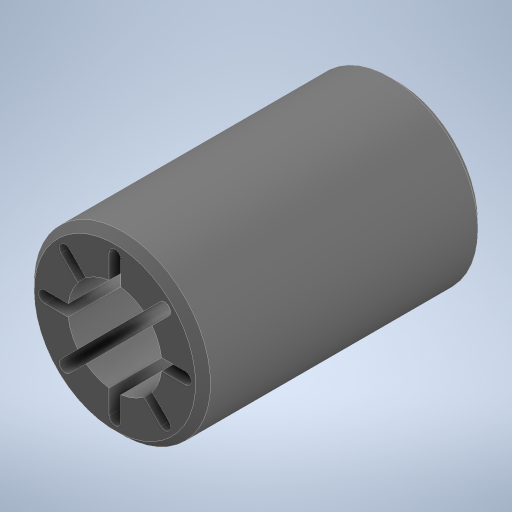
# Autodesk Inventor part: Dry Bearing
Saved by Autodesk Inventor 2023 (Build 270158000, 158)
## iProperties
Created: 2023-02-06
Part Number: Dry Bearing
Material: Generic
Document SubType Name: Modeling
Designer: mbear
Density: 1 g/cm^3
Appearance: Gray
Author: mbear
Autodesk Inventor part; units mm, degrees
ref_plane "YZ Plane" through (0, 0, 0) normal (1, 0, 0) x (0, 1, 0)
ref_plane "XZ Plane" through (0, 0, 0) normal (0, 1, 0) x (-1, 0, 0)
ref_plane "XY Plane" through (0, 0, 0) normal (0, 0, 1) x (1, 0, 0)
sketch "Sketch1" plane through (0, 0, 0) normal (0, 0, 1) x (1, 0, 0)
  circle A0 centre (0, 0) radius 7.5
  circle A1 centre (0, 0) radius 4
  dimension "d0" = 15
  dimension "d1" = 8
  constraints: 2 centre point, 2 coincident
  measures "d0" diameter of A0
  measures "d1" diameter of A1
extrude "Extrusion1" add sketch "Sketch1" along normal blind 24
sketch "Sketch2" plane through (0, 0, 24) normal (0, 0, 1) x (1, 0, 0)
  arc A0 (0.5, 6) -> (-0.5, 6) centre (0, 6) ccw
  line L0 (-0.5, 6) -> (-0.5, 2.6094)
  line L1 (-0.5, 2.6094) -> (0.5, 2.6094)
  line L2 (0.5, 2.6094) -> (0.5, 6)
  line L3 (-4.5962, 3.8891) -> (-2.1987, 1.4916)
  arc A1 (-3.8891, 4.5962) -> (-4.5962, 3.8891) centre (-4.2426, 4.2426) ccw
  line L4 (-1.4916, 2.1987) -> (-3.8891, 4.5962)
  line L5 (-2.1987, 1.4916) -> (-1.4916, 2.1987)
  line L6 (-6, -0.5) -> (-2.6094, -0.5)
  arc A2 (-6, 0.5) -> (-6, -0.5) centre (-6, 0) ccw
  line L7 (-2.6094, 0.5) -> (-6, 0.5)
  line L8 (-2.6094, -0.5) -> (-2.6094, 0.5)
  line L9 (-3.8891, -4.5962) -> (-1.4916, -2.1987)
  arc A3 (-4.5962, -3.8891) -> (-3.8891, -4.5962) centre (-4.2426, -4.2426) ccw
  line L10 (-2.1987, -1.4916) -> (-4.5962, -3.8891)
  line L11 (-1.4916, -2.1987) -> (-2.1987, -1.4916)
  line L12 (0.5, -6) -> (0.5, -2.6094)
  arc A4 (-0.5, -6) -> (0.5, -6) centre (0, -6) ccw
  line L13 (-0.5, -2.6094) -> (-0.5, -6)
  line L14 (0.5, -2.6094) -> (-0.5, -2.6094)
  line L15 (4.5962, -3.8891) -> (2.1987, -1.4916)
  arc A5 (3.8891, -4.5962) -> (4.5962, -3.8891) centre (4.2426, -4.2426) ccw
  line L16 (1.4916, -2.1987) -> (3.8891, -4.5962)
  line L17 (2.1987, -1.4916) -> (1.4916, -2.1987)
  line L18 (6, 0.5) -> (2.6094, 0.5)
  arc A6 (6, -0.5) -> (6, 0.5) centre (6, 0) ccw
  line L19 (2.6094, -0.5) -> (6, -0.5)
  line L20 (2.6094, 0.5) -> (2.6094, -0.5)
  line L21 (3.8891, 4.5962) -> (1.4916, 2.1987)
  arc A7 (4.5962, 3.8891) -> (3.8891, 4.5962) centre (4.2426, 4.2426) ccw
  line L22 (2.1987, 1.4916) -> (4.5962, 3.8891)
  line L23 (1.4916, 2.1987) -> (2.1987, 1.4916)
  point P0 (0, 0)
  dimension "d4" = 1
  dimension "d7" = 360
  constraints: 48 end point, 16 point on circle, 8 centre point, 2 tangent, 1 perpendicular, 1 vertical, 73 other
  measures "d4" diameter of A0
extrude "Extrusion2" cut sketch "Sketch2" against normal blind 24
chamfer "Chamfer1" distance 0.635 angle 45 2 edges at (-7.5, 0, 24) (-7.5, 0, 0)
body "Solid1"
